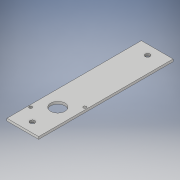
# Autodesk Inventor part: BAG motor top plate
Saved by Autodesk Inventor 2017 (Build 210142000, 142)
## iProperties
Created: 2016-10-01
Part Number: BAG motor top plate
Material: Generic
Document SubType Name: Modeling
Designer: 15102898
Density: 1 g/cm^3
Appearance: Default
Author: 15102898
Autodesk Inventor part; units mm, degrees
ref_plane "YZ Plane" through (0, 0, 0) normal (1, 0, 0) x (0, 1, 0)
ref_plane "XZ Plane" through (0, 0, 0) normal (0, 1, 0) x (-1, 0, 0)
ref_plane "XY Plane" through (0, 0, 0) normal (0, 0, 1) x (1, 0, 0)
sketch "Sketch1" plane through (0, 0, 0) normal (0, 1, 0) x (-1, 0, 0)
  line L0 (0, 0) -> (-42.0116, 0)
  line L1 (-42.0116, 0) -> (-42.0116, -178.054)
  line L2 (-42.0116, -178.054) -> (0, -178.054)
  line L3 (0, -178.054) -> (0, 0)
  circle A0 centre (-21.0058, -12.7) radius 3.175
  circle A1 centre (-21.0058, -165.354) radius 3.175
  circle A2 centre (-3.048, -28.448) radius 2.0193
  circle A3 centre (-38.9636, -64.3636) radius 2.0193
  dimension "d0" = 42.0116
  dimension "d1" = 178.054
  dimension "d2" = 12.7
  dimension "d3" = 12.7
  dimension "d4" = 6.35
  dimension "d5" = 21.0058
  dimension "d6" = 21.0058
  dimension "d7" = 6.35
  dimension "d8" = 28.448
  dimension "d9" = 3.048
  dimension "d10" = 4.0386
  dimension "d11" = 4.0386
  dimension "d12" = 64.3636
  dimension "d13" = 3.048
  constraints: 8 end point, 4 centre point, 2 parallel, 1 horizontal, 1 perpendicular
  measures "d0" distance of L2.end L1.end
  measures "d1" distance of L1.end L0.end
  measures "d2" distance from line of L0 A0.centre
  measures "d3" distance from line of L2 A1.centre
  measures "d4" diameter of A1
  measures "d5" distance from line of L1 A0.centre
  measures "d6" distance from line of L3 A1.centre
  measures "d7" diameter of A0
  measures "d8" distance from line of L0 A2.centre
  measures "d9" distance from line of L3 A2.centre
  measures "d10" diameter of A2
  measures "d11" diameter of A3
  measures "d12" distance from line of L0 A3.centre
  measures "d13" distance from line of L1 A3.centre
extrude "Extrusion1" add sketch "Sketch1" along normal blind 3.175
sketch "Sketch2" plane through (0, 3.175, 0) normal (0, 1, 0) x (1, 0, 0)
  circle A0 centre (21.0058, 46.4058) radius 9.525
  line L0 (0, 178.054) -> (0, 0) projected
  line L1 (0, 0) -> (42.0116, 0) projected
  dimension "d16" = 19.05
  dimension "d17" = 21.0058
  dimension "d18" = 46.4058
  constraints: 1 centre point
  measures "d16" diameter of A0
  measures "d17" distance from line of L0 A0.centre
  measures "d18" distance from line of L1 A0.centre
extrude "Extrusion2" cut sketch "Sketch2" against normal blind 7.9375
body "Solid1"
